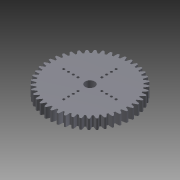
# Autodesk Inventor part: Spur Gear2
Saved by Autodesk Inventor 2014 SP1 (Build 180222100, 222)
## iProperties
Created: 2013-11-19
Part Number: Spur Gear2
Material: Steel
Document SubType Name: Modeling
Designer: jchau3
Categories: <?xml version="1.0" encoding="UTF-16"?> <MemberInstance><Categories><FamilyTemplate><FamilyTemplateParameter ValueType="xs:double" Id="1" ObjectReferenceKey="da_z" ObjectType="kUserParameterObject"/><FamilyTemplateParameter ValueType="xs:double" Id="2" ObjectReferenceKey="da_b" ObjectType="kUserParameterObject"/><FamilyTemplateParameter ValueType="xs:double" Id="3" ObjectReferenceKey="da_beta" ObjectType="kUserParameterObject"/><FamilyTemplateParameter ValueType="xs:double" Id="4" ObjectReferenceKey="da_da" ObjectType="kUserParameterObject"/><FamilyTemplateParameter ValueType="xs:double" Id="5" ObjectReferenceKey="da_aw" ObjectType="kUserParameterObject"/><FamilyTemplateParameter ValueType="xs:string" Id="6" ObjectReferenceKey="EAIAABAAAACIAQAAAAAAAIAAAAAAAAAA" ObjectType="83910656" SubObjectId="SurfaceGeometry"/></FamilyTemplate><ParamToTemplateMap><ParamToTemplate CategoryParameter="//CategoryParameter[@InternalName='046C89C9-8512-4d59-83FE-43B91F4F132A']" TemplateParameter="1"/><ParamToTemplate CategoryParameter="//CategoryParameter[@InternalName='2552DF32-E462-4b46-AEBF-C6C7768E72AC']" TemplateParameter="2"/><ParamToTemplate CategoryParameter="//CategoryParameter[@InternalName='C9EE641D-15FC-4fae-A226-E94C4372FDD7']" TemplateParameter="3"/><ParamToTemplate><ParamToTemplate CategoryParameter="//CategoryParameter[@InternalName='00B6519A-459B-49c7-AD84-2E56D39A5744']" ConstantValue="0.053409"/></ParamToTemplate><ParamToTemplate><ParamToTemplate CategoryParameter="//CategoryParameter[@InternalName='04B31F0E-C7A6-4894-AA32-9629BEFACF47']" ConstantValue="1.000000"/></ParamToTemplate><ParamToTemplate><ParamToTemplate CategoryParameter="//CategoryParameter[@InternalName='43CBEC2E-7847-49e7-A936-2F7889FCB2D9']" ConstantValue="0.250000"/></ParamToTemplate><ParamToTemplate><ParamToTemplate CategoryParameter="//CategoryParameter[@InternalName='B1EFC894-105D-4ebd-86BF-FA20ED196853']" ConstantValue="0.350000"/></ParamToTemplate><ParamToTemplate><ParamToTemplate CategoryParameter="//CategoryParameter[@InternalName='51175063-3D10-4879-93E8-6246FE8B403D']" ConstantValue="2060000000.000000"/></ParamToTemplate><ParamToTemplate><ParamToTemplate CategoryParameter="//CategoryParameter[@InternalName='A3A52E27-4454-46a9-B0BD-C932399B70AF']" ConstantValue="0.300000"/></ParamToTemplate><ParamToTemplate><ParamToTemplate CategoryParameter="//CategoryParameter[@InternalName='91B76062-C214-41d9-B1B9-14D2AB99603D']" ConstantValue="0.112500"/></ParamToTemplate><ParamToTemplate><ParamToTemplate CategoryParameter="//CategoryParameter[@InternalName='374E806E-8B8A-4dda-A9AA-1039D6500AD2']" ConstantValue="8.888889"/></ParamToTemplate><ParamToTemplate><ParamToTemplate CategoryParameter="//CategoryParameter[@InternalName='2D373A89-B862-43d6-8D0B-0CBF12AB9F6C']" ConstantValue="0.349066"/></ParamToTemplate><ParamToTemplate CategoryParameter="//CategoryParameter[@InternalName='37777632-D6A2-4fac-9D53-DB8ACD95C989']" TemplateParameter="4"/><ParamToTemplate CategoryParameter="//CategoryParameter[@InternalName='FD1017F1-B727-4f7e-9707-0F86F1FF9423']" TemplateParameter="5"/><ParamToTemplate><ParamToTemplate CategoryParameter="//CategoryParameter[@InternalName='9E1B4470-B2D3-4ff1-B813-535BB4CDF51A']" ConstantValue="3520000.000000"/></ParamToTemplate><ParamToTemplate><ParamToTemplate CategoryParameter="//CategoryParameter[@InternalName='F8452263-BFF6-458c-9FB1-07C4B99E95CD']" ConstantValue="11400000.000000"/></ParamToTemplate><ParamToTemplate><ParamToTemplate CategoryParameter="//CategoryParameter[@InternalName='3E3BB259-FD49-497f-8171-6EBC954A3479']" ConstantValue="2.000000"/></ParamToTemplate><ParamToTemplate CategoryParameter="//CategoryParameter[@InternalName='27C3BAF2-7550-4e4b-AE2C-0DB134B7D9B7']" TemplateParameter="6"/></ParamToTemplateMap><Category DisplayName="Gear" InternalName="DC85795E-93AB-48d5-8EEE-5A27447B64BD" Mnemonic="Gear"><CategoryParameter DisplayName="z" InternalName="046C89C9-8512-4d59-83FE-43B91F4F132A" Mnemonic="z"/><CategoryParameter DisplayName="b" InternalName="2552DF32-E462-4b46-AEBF-C6C7768E72AC" Mnemonic="b"/><CategoryParameter DisplayName="||b|" InternalName="C9EE641D-15FC-4fae-A226-E94C4372FDD7" Mnemonic="beta"/><CategoryParameter DisplayName="x" InternalName="00B6519A-459B-49c7-AD84-2E56D39A5744" Mnemonic="x"/><CategoryParameter DisplayName="a*" InternalName="04B31F0E-C7A6-4894-AA32-9629BEFACF47" Mnemonic="a"/><CategoryParameter DisplayName="c*" InternalName="43CBEC2E-7847-49e7-A936-2F7889FCB2D9" Mnemonic="c"/><CategoryParameter DisplayName="r|.f|*" InternalName="B1EFC894-105D-4ebd-86BF-FA20ED196853" Mnemonic="rf"/><CategoryParameter DisplayName="E" InternalName="51175063-3D10-4879-93E8-6246FE8B403D" Mnemonic="E"/><CategoryParameter DisplayName="||m|" InternalName="A3A52E27-4454-46a9-B0BD-C932399B70AF" Mnemonic="mi"/><Category DisplayName="SpurGear" InternalName="26C5A22E-A91E-4dfd-A3B3-23CCAFAE1764" Mnemonic="SpurGear"><CategoryParameter DisplayName="m" InternalName="91B76062-C214-41d9-B1B9-14D2AB99603D" Mnemonic="m"/><CategoryParameter DisplayName="P" InternalName="374E806E-8B8A-4dda-A9AA-1039D6500AD2" Mnemonic="PP"/><CategoryParameter DisplayName="||a|" InternalName="2D373A89-B862-43d6-8D0B-0CBF12AB9F6C" Mnemonic="alpha"/><CategoryParameter DisplayName="d|.a|" InternalName="37777632-D6A2-4fac-9D53-DB8ACD95C989" Mnemonic="da"/><CategoryParameter DisplayName="a|.w|" InternalName="FD1017F1-B727-4f7e-9707-0F86F1FF9423" Mnemonic="aw"/><CategoryParameter DisplayName="||s||.Flim|" InternalName="9E1B4470-B2D3-4ff1-B813-535BB4CDF51A" Mnemonic="sFlim"/><CategoryParameter DisplayName="||s||.Hlim|" InternalName="F8452263-BFF6-458c-9FB1-07C4B99E95CD" Mnemonic="sHlim"/><CategoryParameter DisplayName="type" InternalName="3E3BB259-FD49-497f-8171-6EBC954A3479" Mnemonic="type"/><CategoryParameter DisplayName="PitchDiameter" InternalName="27C3BAF2-7550-4e4b-AE2C-0DB134B7D9B7" Mnemonic="IDS_PITCHDIAM"/></Category></Category></Categories></MemberInstance>
Density: 1 g/cm^3
Appearance: Steel
CustomPartVersion: 1
Author: jchau3
Autodesk Inventor part; units mm, degrees
sketch "Sketch1" plane through (0, 0, 0) normal (0, 0, 1) x (1, 0, 0)
  circle A0 centre (0, 0) radius 26.4812
  dimension "d0" = 52.9623
  constraints: 1 centre point
  measures "d0" diameter of A0
extrude "Extrusion1" add sketch "Sketch1" along normal blind 6.35
ref_plane "Work Plane2" through (0, 0, 3.175) normal (0, 0, 1) x (1, 0, 0)
sketch "Sketch2" plane through (0, 0, 0) normal (0, 0, -1) x (-1, 0, 0)
  circle A0 centre (0, 0) radius 26.4812 projected
  circle A1 centre (0, 0) radius 25.5896
  dimension "d3" = 51.1791
  constraints: 1 centre point, 1 coincident
  measures "d3" diameter of A1
surface extrude "Pitch Diameter" sketch "Sketch2" against normal through all shown no curves A1
ref_plane "Work Plane8" through (0, 0, 0) normal (0.9975641, 0.0697565, 0) x (0, 0, 1)
ref_plane "Work Plane9" through (0, 0, 0) normal (1, 0, 0) x (0, 1, 0)
spur gear teeth "Spur Gear" teeth 45 pitch diameter 50.625 tip diameter 52.9623 root diameter 47.9327 face width 6.35 start plane through (0, 0, 0) normal (0, 0, -1) x (-1, 0, 0)
sketch "Sketch3" plane through (0, 0, 6.35) normal (0, 0, 1) x (1, 0, 0)
  arc A0 (-4.1426, 26.1551) -> (-4.573, 23.526) centre (8.3362, 22.7624) ccw projected
  arc A1 (-4.573, 23.526) -> (-5.3913, 23.3521) centre (0, 0) ccw projected
  arc A2 (-5.3913, 23.3521) -> (-6.8538, 25.5788) centre (-16.8738, 17.4038) ccw projected
  arc A3 (-6.8538, 25.5788) -> (-7.7423, 25.3241) centre (0, 0) ccw projected
  arc A4 (-7.7423, 25.3241) -> (-7.8027, 22.6606) centre (5.0872, 23.701) ccw projected
  arc A5 (-7.8027, 22.6606) -> (-8.5888, 22.3745) centre (0, 0) ccw projected
  arc A6 (-8.5888, 22.3745) -> (-10.347, 24.376) centre (-19.1317, 14.8861) ccw projected
  arc A7 (-10.347, 24.376) -> (-11.1914, 24.0001) centre (0, 0) ccw projected
  arc A8 (-11.1914, 24.0001) -> (-10.8805, 21.3542) centre (1.7391, 24.1784) ccw projected
  arc A9 (-10.8805, 21.3542) -> (-11.6191, 20.9614) centre (0, 0) ccw projected
  arc A10 (-11.6191, 20.9614) -> (-13.6388, 22.6988) centre (-21.0173, 12.0786) ccw projected
  arc A11 (-13.6388, 22.6988) -> (-14.4227, 22.209) centre (0, 0) ccw projected
  arc A12 (-14.4227, 22.209) -> (-13.7465, 19.6321) centre (-1.6428, 24.1851) ccw projected
  arc A13 (-13.7465, 19.6321) -> (-14.4233, 19.1404) centre (0, 0) ccw projected
  arc A14 (-14.4233, 19.1404) -> (-16.6651, 20.5797) centre (-22.4938, 9.036) ccw projected
  arc A15 (-16.6651, 20.5797) -> (-17.3732, 19.9856) centre (0, 0) ccw projected
  arc A16 (-17.3732, 19.9856) -> (-16.345, 17.5279) centre (-4.9927, 23.7211) ccw projected
  arc A17 (-16.345, 17.5279) -> (-16.9468, 16.9468) centre (0, 0) ccw projected
  arc A18 (-16.9468, 16.9468) -> (-19.3671, 18.0601) centre (-23.5324, 5.8175) ccw projected
  arc A19 (-19.3671, 18.0601) -> (-19.9856, 17.3732) centre (0, 0) ccw projected
  arc A20 (-19.9856, 17.3732) -> (-18.6253, 15.0825) centre (-8.2455, 22.7954) ccw projected
  arc A21 (-18.6253, 15.0825) -> (-19.1404, 14.4233) centre (0, 0) ccw projected
  arc A22 (-19.1404, 14.4233) -> (-21.6921, 15.189) centre (-24.113, 2.4858) ccw projected
  arc A23 (-21.6921, 15.189) -> (-22.209, 14.4227) centre (0, 0) ccw projected
  arc A24 (-22.209, 14.4227) -> (-20.5432, 12.3436) centre (-11.3377, 21.426) ccw projected
  arc A25 (-20.5432, 12.3436) -> (-20.9614, 11.6191) centre (0, 0) ccw projected
  arc A26 (-20.9614, 11.6191) -> (-23.5949, 12.0222) centre (-24.2243, -0.8943) ccw projected
  arc A27 (-23.5949, 12.0222) -> (-24.0001, 11.1914) centre (0, 0) ccw projected
  arc A28 (-24.0001, 11.1914) -> (-22.0611, 9.3644) centre (-14.2093, 19.6396) ccw projected
  arc A29 (-22.0611, 9.3644) -> (-22.3745, 8.5888) centre (0, 0) ccw projected
  arc A30 (-22.3745, 8.5888) -> (-25.0384, 8.6214) centre (-23.8641, -4.2569) ccw projected
  arc A31 (-25.0384, 8.6214) -> (-25.3241, 7.7423) centre (0, 0) ccw projected
  arc A32 (-25.3241, 7.7423) -> (-23.1497, 6.2029) centre (-16.8043, 17.4709) ccw projected
  arc A33 (-23.1497, 6.2029) -> (-23.3521, 5.3913) centre (0, 0) ccw projected
  arc A34 (-23.3521, 5.3913) -> (-25.9946, 5.0528) centre (-23.0394, -7.5367) ccw projected
  arc A35 (-25.9946, 5.0528) -> (-26.1551, 4.1426) centre (0, 0) ccw projected
  arc A36 (-26.1551, 4.1426) -> (-23.7877, 2.9208) centre (-19.0723, 14.9622) ccw projected
  arc A37 (-23.7877, 2.9208) -> (-23.8751, 2.0888) centre (0, 0) ccw projected
  arc A38 (-23.8751, 2.0888) -> (-26.4449, 1.3859) centre (-21.7663, -10.6699) ccw projected
  arc A39 (-26.4449, 1.3859) -> (-26.4771, 0.4622) centre (0, 0) ccw projected
  arc A40 (-26.4771, 0.4622) -> (-23.9627, -0.4183) centre (-20.969, 12.1622) ccw projected
  arc A41 (-23.9627, -0.4183) -> (-23.9335, -1.2543) centre (0, 0) ccw projected
  arc A42 (-23.9335, -1.2543) -> (-26.3804, -2.308) centre (-20.0695, -13.5953) ccw projected
  arc A43 (-26.3804, -2.308) -> (-26.2838, -3.2272) centre (0, 0) ccw projected
  arc A44 (-26.2838, -3.2272) -> (-23.6713, -3.7492) centre (-22.4576, 9.1255) ccw projected
  arc A45 (-23.6713, -3.7492) -> (-23.526, -4.573) centre (0, 0) ccw projected
  arc A46 (-23.526, -4.573) -> (-25.8025, -5.957) centre (-17.9821, -16.2561) ccw projected
  arc A47 (-25.8025, -5.957) -> (-25.5788, -6.8538) centre (0, 0) ccw projected
  arc A48 (-25.5788, -6.8538) -> (-22.9191, -7.0071) centre (-23.5091, 5.9112) ccw projected
  arc A49 (-22.9191, -7.0071) -> (-22.6606, -7.8027) centre (0, 0) ccw projected
  arc A50 (-22.6606, -7.8027) -> (-24.7223, -9.49) centre (-15.5447, -18.6006) ccw projected
  arc A51 (-24.7223, -9.49) -> (-24.376, -10.347) centre (0, 0) ccw projected
  arc A52 (-24.376, -10.347) -> (-21.7209, -10.1286) centre (-24.103, 2.5819) ccw projected
  arc A53 (-21.7209, -10.1286) -> (-21.3542, -10.8805) centre (0, 0) ccw projected
  arc A54 (-21.3542, -10.8805) -> (-23.1609, -12.8383) centre (-12.8047, -20.583) ccw projected
  arc A55 (-23.1609, -12.8383) -> (-22.6988, -13.6388) centre (0, 0) ccw projected
  arc A56 (-22.6988, -13.6388) -> (-20.0999, -13.053) centre (-24.2277, -0.7977) ccw projected
  arc A57 (-20.0999, -13.053) -> (-19.6321, -13.7465) centre (0, 0) ccw projected
  arc A58 (-19.6321, -13.7465) -> (-21.1488, -15.9368) centre (-9.8155, -22.1647) ccw projected
  arc A59 (-21.1488, -15.9368) -> (-20.5797, -16.6651) centre (0, 0) ccw projected
  arc A60 (-20.5797, -16.6651) -> (-18.0876, -15.7233) centre (-23.8809, -4.1618) ccw projected
  arc A61 (-18.0876, -15.7233) -> (-17.5279, -16.345) centre (0, 0) ccw projected
  arc A62 (-17.5279, -16.345) -> (-18.725, -18.725) centre (-6.6352, -23.3151) ccw projected
  arc A63 (-18.725, -18.725) -> (-18.0601, -19.3671) centre (0, 0) ccw projected
  arc A64 (-18.0601, -19.3671) -> (-15.7233, -18.0876) centre (-23.0693, -7.4449) ccw projected
  arc A65 (-15.7233, -18.0876) -> (-15.0825, -18.6253) centre (0, 0) ccw projected
  arc A66 (-15.0825, -18.6253) -> (-15.9368, -21.1488) centre (-3.3258, -24.0116) ccw projected
  arc A67 (-15.9368, -21.1488) -> (-15.189, -21.6921) centre (0, 0) ccw projected
  arc A68 (-15.189, -21.6921) -> (-13.053, -20.0999) centre (-21.8087, -10.5831) ccw projected
  arc A69 (-13.053, -20.0999) -> (-12.3436, -20.5432) centre (0, 0) ccw projected
  arc A70 (-12.3436, -20.5432) -> (-12.8383, -23.1609) centre (0.0483, -24.2408) ccw projected
  arc A71 (-12.8383, -23.1609) -> (-12.0222, -23.5949) centre (0, 0) ccw projected
  arc A72 (-12.0222, -23.5949) -> (-10.1286, -21.7209) centre (-20.1235, -13.5152) ccw projected
  arc A73 (-10.1286, -21.7209) -> (-9.3644, -22.0611) centre (0, 0) ccw projected
  arc A74 (-9.3644, -22.0611) -> (-9.49, -24.7223) centre (3.4215, -23.9982) ccw projected
  arc A75 (-9.49, -24.7223) -> (-8.6214, -25.0384) centre (0, 0) ccw projected
  arc A76 (-8.6214, -25.0384) -> (-7.0071, -22.9191) centre (-18.0467, -16.1844) ccw projected
  arc A77 (-7.0071, -22.9191) -> (-6.2029, -23.1497) centre (0, 0) ccw projected
  arc A78 (-6.2029, -23.1497) -> (-5.957, -25.8025) centre (6.7281, -23.2884) ccw projected
  arc A79 (-5.957, -25.8025) -> (-5.0528, -25.9946) centre (0, 0) ccw projected
  arc A80 (-5.0528, -25.9946) -> (-3.7492, -23.6713) centre (-15.6187, -18.5385) ccw projected
  arc A81 (-3.7492, -23.6713) -> (-2.9208, -23.7877) centre (0, 0) ccw projected
  arc A82 (-2.9208, -23.7877) -> (-2.308, -26.3804) centre (9.9037, -22.1254) ccw projected
  arc A83 (-2.308, -26.3804) -> (-1.3859, -26.4449) centre (0, 0) ccw projected
  arc A84 (-1.3859, -26.4449) -> (-0.4183, -23.9627) centre (-12.8866, -20.5318) ccw projected
  arc A85 (-0.4183, -23.9627) -> (0.4183, -23.9627) centre (0, 0) ccw projected
  arc A86 (0.4183, -23.9627) -> (1.3859, -26.4449) centre (12.8866, -20.5318) ccw projected
  arc A87 (1.3859, -26.4449) -> (2.308, -26.3804) centre (0, 0) ccw projected
  arc A88 (2.308, -26.3804) -> (2.9208, -23.7877) centre (-9.9037, -22.1254) ccw projected
  arc A89 (2.9208, -23.7877) -> (3.7492, -23.6713) centre (0, 0) ccw projected
  arc A90 (3.7492, -23.6713) -> (5.0528, -25.9946) centre (15.6187, -18.5385) ccw projected
  arc A91 (5.0528, -25.9946) -> (5.957, -25.8025) centre (0, 0) ccw projected
  arc A92 (5.957, -25.8025) -> (6.2029, -23.1497) centre (-6.7281, -23.2884) ccw projected
  arc A93 (6.2029, -23.1497) -> (7.0071, -22.9191) centre (0, 0) ccw projected
  arc A94 (7.0071, -22.9191) -> (8.6214, -25.0384) centre (18.0467, -16.1844) ccw projected
  arc A95 (8.6214, -25.0384) -> (9.49, -24.7223) centre (0, 0) ccw projected
  arc A96 (9.49, -24.7223) -> (9.3644, -22.0611) centre (-3.4215, -23.9982) ccw projected
  arc A97 (9.3644, -22.0611) -> (10.1286, -21.7209) centre (0, 0) ccw projected
  arc A98 (10.1286, -21.7209) -> (12.0222, -23.5949) centre (20.1235, -13.5152) ccw projected
  arc A99 (12.0222, -23.5949) -> (12.8383, -23.1609) centre (0, 0) ccw projected
  arc A100 (12.8383, -23.1609) -> (12.3436, -20.5432) centre (-0.0483, -24.2408) ccw projected
  arc A101 (12.3436, -20.5432) -> (13.053, -20.0999) centre (0, 0) ccw projected
  arc A102 (13.053, -20.0999) -> (15.189, -21.6921) centre (21.8087, -10.5831) ccw projected
  arc A103 (15.189, -21.6921) -> (15.9368, -21.1488) centre (0, 0) ccw projected
  arc A104 (15.9368, -21.1488) -> (15.0825, -18.6253) centre (3.3258, -24.0116) ccw projected
  arc A105 (15.0825, -18.6253) -> (15.7233, -18.0876) centre (0, 0) ccw projected
  arc A106 (15.7233, -18.0876) -> (18.0601, -19.3671) centre (23.0693, -7.4449) ccw projected
  arc A107 (18.0601, -19.3671) -> (18.725, -18.725) centre (0, 0) ccw projected
  arc A108 (18.725, -18.725) -> (17.5279, -16.345) centre (6.6352, -23.3151) ccw projected
  arc A109 (17.5279, -16.345) -> (18.0876, -15.7233) centre (0, 0) ccw projected
  arc A110 (18.0876, -15.7233) -> (20.5797, -16.6651) centre (23.8809, -4.1618) ccw projected
  arc A111 (20.5797, -16.6651) -> (21.1488, -15.9368) centre (0, 0) ccw projected
  arc A112 (21.1488, -15.9368) -> (19.6321, -13.7465) centre (9.8155, -22.1647) ccw projected
  arc A113 (19.6321, -13.7465) -> (20.0999, -13.053) centre (0, 0) ccw projected
  arc A114 (20.0999, -13.053) -> (22.6988, -13.6388) centre (24.2277, -0.7977) ccw projected
  arc A115 (22.6988, -13.6388) -> (23.1609, -12.8383) centre (0, 0) ccw projected
  arc A116 (23.1609, -12.8383) -> (21.3542, -10.8805) centre (12.8047, -20.583) ccw projected
  arc A117 (21.3542, -10.8805) -> (21.7209, -10.1286) centre (0, 0) ccw projected
  arc A118 (21.7209, -10.1286) -> (24.376, -10.347) centre (24.103, 2.5819) ccw projected
  arc A119 (24.376, -10.347) -> (24.7223, -9.49) centre (0, 0) ccw projected
  arc A120 (24.7223, -9.49) -> (22.6606, -7.8027) centre (15.5447, -18.6006) ccw projected
  arc A121 (22.6606, -7.8027) -> (22.9191, -7.0071) centre (0, 0) ccw projected
  arc A122 (22.9191, -7.0071) -> (25.5788, -6.8538) centre (23.5091, 5.9112) ccw projected
  arc A123 (25.5788, -6.8538) -> (25.8025, -5.957) centre (0, 0) ccw projected
  arc A124 (25.8025, -5.957) -> (23.526, -4.573) centre (17.9821, -16.2561) ccw projected
  arc A125 (23.526, -4.573) -> (23.6713, -3.7492) centre (0, 0) ccw projected
  arc A126 (23.6713, -3.7492) -> (26.2838, -3.2272) centre (22.4576, 9.1255) ccw projected
  arc A127 (26.2838, -3.2272) -> (26.3804, -2.308) centre (0, 0) ccw projected
  arc A128 (26.3804, -2.308) -> (23.9335, -1.2543) centre (20.0695, -13.5953) ccw projected
  arc A129 (23.9335, -1.2543) -> (23.9627, -0.4183) centre (0, 0) ccw projected
  arc A130 (23.9627, -0.4183) -> (26.4771, 0.4622) centre (20.969, 12.1622) ccw projected
  arc A131 (26.4771, 0.4622) -> (26.4449, 1.3859) centre (0, 0) ccw projected
  arc A132 (26.4449, 1.3859) -> (23.8751, 2.0888) centre (21.7663, -10.6699) ccw projected
  arc A133 (23.8751, 2.0888) -> (23.7877, 2.9208) centre (0, 0) ccw projected
  arc A134 (23.7877, 2.9208) -> (26.1551, 4.1426) centre (19.0723, 14.9622) ccw projected
  arc A135 (26.1551, 4.1426) -> (25.9946, 5.0528) centre (0, 0) ccw projected
  arc A136 (25.9946, 5.0528) -> (23.3521, 5.3913) centre (23.0394, -7.5367) ccw projected
  arc A137 (23.3521, 5.3913) -> (23.1497, 6.2029) centre (0, 0) ccw projected
  arc A138 (23.1497, 6.2029) -> (25.3241, 7.7423) centre (16.8043, 17.4709) ccw projected
  arc A139 (25.3241, 7.7423) -> (25.0384, 8.6214) centre (0, 0) ccw projected
  arc A140 (25.0384, 8.6214) -> (22.3745, 8.5888) centre (23.8641, -4.2569) ccw projected
  arc A141 (22.3745, 8.5888) -> (22.0611, 9.3644) centre (0, 0) ccw projected
  arc A142 (22.0611, 9.3644) -> (24.0001, 11.1914) centre (14.2093, 19.6396) ccw projected
  arc A143 (24.0001, 11.1914) -> (23.5949, 12.0222) centre (0, 0) ccw projected
  arc A144 (23.5949, 12.0222) -> (20.9614, 11.6191) centre (24.2243, -0.8943) ccw projected
  arc A145 (20.9614, 11.6191) -> (20.5432, 12.3436) centre (0, 0) ccw projected
  arc A146 (20.5432, 12.3436) -> (22.209, 14.4227) centre (11.3377, 21.426) ccw projected
  arc A147 (22.209, 14.4227) -> (21.6921, 15.189) centre (0, 0) ccw projected
  arc A148 (21.6921, 15.189) -> (19.1404, 14.4233) centre (24.113, 2.4858) ccw projected
  arc A149 (19.1404, 14.4233) -> (18.6253, 15.0825) centre (0, 0) ccw projected
  arc A150 (18.6253, 15.0825) -> (19.9856, 17.3732) centre (8.2455, 22.7954) ccw projected
  arc A151 (19.9856, 17.3732) -> (19.3671, 18.0601) centre (0, 0) ccw projected
  arc A152 (19.3671, 18.0601) -> (16.9468, 16.9468) centre (23.5324, 5.8175) ccw projected
  arc A153 (16.9468, 16.9468) -> (16.345, 17.5279) centre (0, 0) ccw projected
  arc A154 (16.345, 17.5279) -> (17.3732, 19.9856) centre (4.9927, 23.7211) ccw projected
  arc A155 (17.3732, 19.9856) -> (16.6651, 20.5797) centre (0, 0) ccw projected
  arc A156 (16.6651, 20.5797) -> (14.4233, 19.1404) centre (22.4938, 9.036) ccw projected
  arc A157 (14.4233, 19.1404) -> (13.7465, 19.6321) centre (0, 0) ccw projected
  arc A158 (13.7465, 19.6321) -> (14.4227, 22.209) centre (1.6428, 24.1851) ccw projected
  arc A159 (14.4227, 22.209) -> (13.6388, 22.6988) centre (0, 0) ccw projected
  arc A160 (13.6388, 22.6988) -> (11.6191, 20.9614) centre (21.0173, 12.0786) ccw projected
  arc A161 (11.6191, 20.9614) -> (10.8805, 21.3542) centre (0, 0) ccw projected
  arc A162 (10.8805, 21.3542) -> (11.1914, 24.0001) centre (-1.7391, 24.1784) ccw projected
  arc A163 (11.1914, 24.0001) -> (10.347, 24.376) centre (0, 0) ccw projected
  arc A164 (10.347, 24.376) -> (8.5888, 22.3745) centre (19.1317, 14.8861) ccw projected
  arc A165 (8.5888, 22.3745) -> (7.8027, 22.6606) centre (0, 0) ccw projected
  arc A166 (7.8027, 22.6606) -> (7.7423, 25.3241) centre (-5.0872, 23.701) ccw projected
  arc A167 (7.7423, 25.3241) -> (6.8538, 25.5788) centre (0, 0) ccw projected
  arc A168 (6.8538, 25.5788) -> (5.3913, 23.3521) centre (16.8738, 17.4038) ccw projected
  arc A169 (5.3913, 23.3521) -> (4.573, 23.526) centre (0, 0) ccw projected
  arc A170 (4.573, 23.526) -> (4.1426, 26.1551) centre (-8.3362, 22.7624) ccw projected
  arc A171 (4.1426, 26.1551) -> (3.2272, 26.2838) centre (0, 0) ccw projected
  arc A172 (3.2272, 26.2838) -> (2.0888, 23.8751) centre (14.2875, 19.5828) ccw projected
  arc A173 (2.0888, 23.8751) -> (1.2543, 23.9335) centre (0, 0) ccw projected
  arc A174 (1.2543, 23.9335) -> (0.4622, 26.4771) centre (-11.423, 21.3807) ccw projected
  arc A175 (0.4622, 26.4771) -> (-0.4622, 26.4771) centre (0, 0) ccw projected
  arc A176 (-0.4622, 26.4771) -> (-1.2543, 23.9335) centre (11.423, 21.3807) ccw projected
  arc A177 (-1.2543, 23.9335) -> (-2.0888, 23.8751) centre (0, 0) ccw projected
  arc A178 (-2.0888, 23.8751) -> (-3.2272, 26.2838) centre (-14.2875, 19.5828) ccw projected
  arc A179 (-3.2272, 26.2838) -> (-4.1426, 26.1551) centre (0, 0) ccw projected
  circle A180 centre (0, 0) radius 3
  circle A181 centre (7.5, 0) radius 0.75
  circle A182 centre (10.5, 0) radius 0.75
  circle A183 centre (13.5, 0) radius 0.75
  circle A184 centre (16.5, 0) radius 0.75
  circle A185 centre (0, 7.5) radius 0.75
  circle A186 centre (0, 10.5) radius 0.75
  circle A187 centre (0, 13.5) radius 0.75
  circle A188 centre (0, 16.5) radius 0.75
  circle A189 centre (-7.5, 0) radius 0.75
  circle A190 centre (-10.5, 0) radius 0.75
  circle A191 centre (-13.5, 0) radius 0.75
  circle A192 centre (-16.5, 0) radius 0.75
  circle A193 centre (0, -7.5) radius 0.75
  circle A194 centre (0, -10.5) radius 0.75
  circle A195 centre (0, -13.5) radius 0.75
  circle A196 centre (0, -16.5) radius 0.75
  dimension "d49" = 6
  dimension "d50" = 1.5
  dimension "d51" = 7.5
  dimension "d52" = 1.5
  dimension "d53" = 3
  dimension "d54" = 3
  dimension "d55" = 3
  dimension "d58" = 360
  constraints: 17 centre point, 1 coincident, 33 other
  measures "d49" diameter of A180
  measures "d50" diameter of A181
  measures "d51" distance of A181.centre A1.centre
  measures "d52" diameter of A182
  measures "d53" distance of A182.centre A181.centre
  measures "d54" distance of A183.centre A182.centre
  measures "d55" distance of A184.centre A183.centre
extrude "Extrusion2" cut sketch "Sketch3" against normal through all keep common part
equation "\"d0\" = da_da"
equation "\"d1\" = da_b"
equation "\"d3\" = da_dw"
equation "\"d16\" = da_aw"
equation "\"d43\" = da_aw"
equation "\"d46\" = da_aw"
equation "\"da_da\" = 52.962323"
equation "\"da_b\" = 6.35"
equation "\"da_dw\" = 51.179104"
equation "\"da_aw\" = 38.1"
body "Solid1"
body "Srf1"
